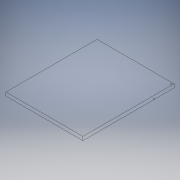
# Autodesk Inventor part: Horizontal Shelf
Saved by Autodesk Inventor 2016 (Build 200138000, 138)
## iProperties
Created: 2017-10-30
Part Number: Horizontal Shelf
Material: Generic
Document SubType Name: Modeling
Designer: mathaetaes
Density: 1 g/cm^3
Appearance: Default
Author: mathaetaes
Autodesk Inventor part; units mm, degrees
ref_plane "YZ Plane" through (0, 0, 0) normal (1, 0, 0) x (0, 1, 0)
ref_plane "XZ Plane" through (0, 0, 0) normal (0, 1, 0) x (-1, 0, 0)
ref_plane "XY Plane" through (0, 0, 0) normal (0, 0, 1) x (1, 0, 0)
sketch "Sketch1" plane through (0, 0, 0) normal (0, 1, 0) x (-1, 0, 0)
  line L0 (198.4375, -234.95) -> (-198.4375, -234.95)
  line L1 (-198.4375, -234.95) -> (-198.4375, 234.95)
  line L2 (-198.4375, 234.95) -> (198.4375, 234.95)
  line L3 (198.4375, 234.95) -> (198.4375, -234.95)
  line L4 (0, -328.93) -> (0, 328.93) projected
  line L5 (277.8125, 0) -> (-277.8125, 0) projected
  point P0 (0, 0)
  dimension "d0" = 396.875
  dimension "d1" = 469.9
  dimension "d4" = 198.4375
  dimension "d8" = 234.95
  constraints: 8 end point, 2 parallel, 1 horizontal, 1 perpendicular
  measures "d0" distance of L1.end L2.end
  measures "d1" distance of L0.end L1.end
  measures "d4" distance between parallel lines of L3 L4
  measures "d8" distance between parallel lines of L5 L0
extrude "Board" add sketch "Sketch1" along normal blind 19.05
sketch "Sketch3" plane through (0, 0, 0) normal (0, -1, 0) x (1, 0, 0)
  circle A0 centre (193.675, -219.075) radius 3.175
  line L0 (-198.4375, -234.95) -> (198.4375, -234.95) projected
  line L1 (198.4375, -234.95) -> (198.4375, 234.95) projected
  point P0 (0, 0)
  dimension "d19" = 6.35
  dimension "d22" = 12.7
  dimension "d23" = 1.5875
  constraints: 1 centre point
  measures "d19" diameter of A0
  measures "d22" distance edge to line of A0 L0
  measures "d23" distance edge to line of A0 L1
extrude "Wire Hole" cut sketch "Sketch3" against normal blind 19.05
sketch "Sketch4" plane through (0, 0, 0) normal (0, -1, 0) x (1, 0, 0)
  line L0 (-198.4375, -127) -> (198.4375, -127)
  line L1 (198.4375, -127) -> (198.4375, -133.35)
  line L2 (198.4375, -133.35) -> (-198.4375, -133.35)
  line L3 (-198.4375, -133.35) -> (-198.4375, -127)
  line L4 (-198.4375, -234.95) -> (198.4375, -234.95) projected
  line L5 (-198.4375, 234.95) -> (-198.4375, -234.95) projected
  line L6 (198.4375, -234.95) -> (198.4375, 234.95) projected
  point P0 (0, 0)
  point P1 (192.0875, -244.475)
  point P2 (198.4375, -231.775)
  dimension "d15" = 6.35
  dimension "d16" = 101.6
  constraints: 8 end point, 2 collinear, 2 parallel, 1 horizontal, 1 perpendicular, 1 other
  measures "d15" distance of L0.end L1.end
extrude "Wine Rack Backing Dado" cut sketch "Sketch4" against normal blind 6.35 contours L0 L1 L2 L3
equation "\"d4\" = 0.5 * d0"
equation "\"d8\" = 0.5 * d1"
body "Solid1"
